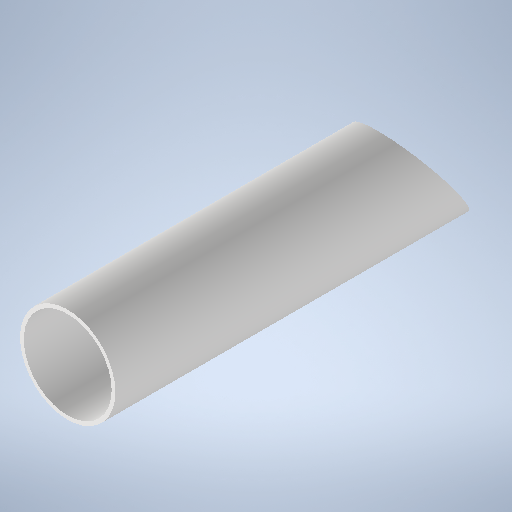
# Autodesk Inventor part: МОО 068 ракета труба 8
Saved by Autodesk Inventor 2025 (Build 290162010, 162A)
## iProperties
Created: 2024-05-24
Part Number: МОО 068 ракета труба 8
Material: Stainless Steel
Document SubType Name: Modeling
Designer: admin
Density: 8 g/cm^3
Appearance: Default
Author: admin
Autodesk Inventor part; units mm, degrees
ref_plane "YZ Plane" through (0, 0, 0) normal (1, 0, 0) x (0, 1, 0)
ref_plane "XZ Plane" through (0, 0, 0) normal (0, 1, 0) x (-1, 0, 0)
ref_plane "XY Plane" through (0, 0, 0) normal (0, 0, 1) x (1, 0, 0)
sketch "Sketch1" plane through (0, 0, 0) normal (0, 0, 1) x (1, 0, 0)
  circle A0 centre (0, 0) radius 38
  circle A1 centre (0, 0) radius 35
  dimension "d0" = 76
  dimension "d1" = 3
  constraints: 2 centre point, 1 coincident
  measures "d0" diameter of A0
  measures "d1" radial gap between concentric circles of A0 A1
extrude "Extrusion1" add sketch "Sketch1" along normal blind 300
sketch "Sketch2" plane through (0, 0, 0) normal (1, 0, 0) x (0, 1, 0)
  line L0 (38, 300) -> (-38, 300) projected
  line L1 (38, 0) -> (-38, 0) projected
  line L2 (-38, 0) -> (38, 53.2158)
  line L3 (38, 53.2158) -> (38, 0)
  line L4 (38, 0) -> (38, 300) projected
  point P0 (0, 0)
  dimension "d4" = 35
  constraints: 4 end point, 1 collinear
  measures "d4" angle of L2 L1
extrude "Extrusion2" cut sketch "Sketch2" along normal mid plane 300
body "Solid1"
